# Autodesk Inventor part: intersection_extension
Saved by Autodesk Inventor 2021 (Build 250183000, 183)
## iProperties
Created: 2021-01-02
Part Number: intersection_extension
Material: Generic
Document SubType Name: Modeling
Designer: Tomasz
Density: 1 g/cm^3
Appearance: Default
Author: Tomasz
Autodesk Inventor part; units mm, degrees
ref_plane "YZ Plane" through (0, 0, 0) normal (1, 0, 0) x (0, 1, 0)
ref_plane "XZ Plane" through (0, 0, 0) normal (0, 1, 0) x (-1, 0, 0)
ref_plane "XY Plane" through (0, 0, 0) normal (0, 0, 1) x (1, 0, 0)
sketch "Sketch1" plane through (0, 0, 0) normal (0, 1, 0) x (-1, 0, 0)
  line L0 (170, 275) -> (0, 275)
  line L1 (0, 275) -> (0, -275)
  line L2 (0, -275) -> (170, -275)
  line L3 (170, -275) -> (170, 275)
  line L4 (170, 255) -> (0, 255)
  line L5 (170, -255) -> (0, -255)
  point P0 (0, 0)
  point P1 (0, 0)
  dimension "d0" = 170
  dimension "d1" = 550
  dimension "d4" = 20
  dimension "d5" = 20
  constraints: 12 end point, 4 point on line, 3 perpendicular, 2 parallel, 1 coincident, 1 horizontal, 1 midpoint
  measures "d0" distance of L0.start L0.end
  measures "d1" distance of L2.end L0.start
  measures "d4" distance between parallel lines of L0 L4
  measures "d5" distance between parallel lines of L2 L5
extrude "Extrusion1" add sketch "Sketch1" along normal blind 3
extrude "Extrusion2" add sketch "Sketch1" along normal blind 3.1 contours L3 L4 L1 L0 | L3 L2 L1 L5
equation "\"d1\" = track_width"
equation "\"d4\" = curb_width"
equation "\"d5\" = curb_width"
equation "\"d2\" = track_height"
equation "\"d6\" = track_height + curb_height"
equation "\"track_width\" = 550"
equation "\"curb_width\" = 20"
equation "\"track_height\" = 3"
equation "\"curb_height\" = 0.1"
body "Solid1"
